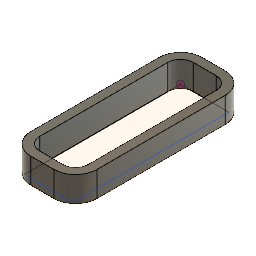
AidanSafeHandle (Autodesk Fusion 360 design; units mm, degrees)
Autodesk Fusion 360 part; units mm, degrees
sketch "Sketch1" plane through (0, 0, 0) normal (0, 1, 0) x (1, 0, 0)
  line L0 (10, 0) -> (25.2572, 0)
  line L1 (0, 0) -> (28.18, 0)
  line L2 (38.18, -10) -> (38.18, -111.08)
  line L3 (28.18, -121.08) -> (10, -121.08)
  line L4 (0, -111.08) -> (0, -10)
  arc A0 (28.18, -121.08) -> (38.18, -111.08) centre (28.18, -111.08) ccw
  arc A1 (0, -111.08) -> (10, -121.08) centre (10, -111.08) ccw
  arc A2 (10, 0) -> (0, -10) centre (10, -10) ccw
  arc A3 (38.18, -10) -> (28.18, 0) centre (28.18, -10) ccw
  line L5 (0, 7) -> (10, 7)
  line L6 (10, 7) -> (25.2572, 7)
  line L7 (25.2572, 7) -> (28.18, 7)
  arc A4 (45.18, -10) -> (28.18, 7) centre (28.18, -10) ccw
  line L8 (45.18, -10) -> (45.18, -111.08)
  arc A5 (28.18, -128.08) -> (45.18, -111.08) centre (28.18, -111.08) ccw
  line L9 (28.18, -128.08) -> (10, -128.08)
  arc A6 (-7, -111.08) -> (10, -128.08) centre (10, -111.08) ccw
  line L10 (-7, -111.08) -> (-7, -10)
  arc A7 (10, 7) -> (-7, -10) centre (10, -10) ccw
  dimension "d1" = 121.08
  dimension "d2" = 38.18
  dimension "d3" = 10
  dimension "d4" = 10
  dimension "d5" = 7
  measures "d3" radius of A0
  measures "d4" radius of A3
extrude "Extrude1" add sketch "Sketch1" along normal blind 20
sketch "Sketch2" plane through (0, 0, 0) normal (0, -1, 0) x (1, 0, 0)
  arc A0 (38.18, 111.08) -> (28.18, 121.08) centre (28.18, 111.08) ccw
  line L0 (38.18, 111.08) -> (38.18, 10)
  arc A1 (28.18, 0) -> (38.18, 10) centre (28.18, 10) ccw
  line L1 (28.18, 0) -> (10, 0)
  arc A2 (0, 10) -> (10, 0) centre (10, 10) ccw
  line L2 (0, 10) -> (0, 111.08)
  arc A3 (10, 121.08) -> (0, 111.08) centre (10, 111.08) ccw
  line L3 (10, 121.08) -> (28.18, 121.08)
  line L4 (10, -7) -> (28.18, -7)
  arc A4 (28.18, -7) -> (45.18, 10) centre (28.18, 10) ccw
  line L5 (45.18, 10) -> (45.18, 111.08)
  arc A5 (45.18, 111.08) -> (28.18, 128.08) centre (28.18, 111.08) ccw
  line L6 (28.18, 128.08) -> (10, 128.08)
  arc A6 (10, 128.08) -> (-7, 111.08) centre (10, 111.08) ccw
  line L7 (-7, 111.08) -> (-7, 10)
  arc A7 (-7, 10) -> (10, -7) centre (10, 10) ccw
  line L8 (0, 0) -> (38.18, 0)
  line L9 (38.18, 0) -> (38.18, 123.1008)
  line L10 (38.18, 123.1008) -> (0, 123.1008)
  line L11 (0, 123.1008) -> (0, 0)
